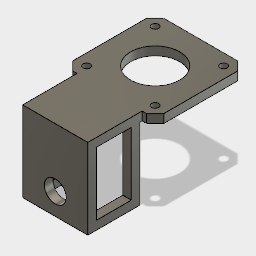
Stepper v4 (Autodesk Fusion 360 design; units mm, degrees)
Autodesk Fusion 360 part; units mm, degrees
note: some values were not read from the file. Set by a fixed rule: which face or edge a step refers to.
sketch "Sketch1" plane through (0, 0, 0) normal (0, 1, 0) x (1, 0, 0)
  line L0 (0, 0) -> (42, 0)
  line L1 (42, 0) -> (42, -42)
  line L2 (42, -42) -> (0, -42)
  line L3 (0, -42) -> (0, 0)
  dimension "d1" = 42
  dimension "d2" = 42
  measures "d1" distance of L0.start L2.end
  measures "d2" distance of L0.start L0.end
extrude "Extrude1" add sketch "Sketch1" along normal blind 33 makes body 1
sketch "Sketch2" plane through (0, 33, 0) normal (0, 1, 0) x (-1, 0, 0)
  line L0 (0, 42) -> (-42, 42)
  line L1 (-42, 42) -> (-42, 0)
  line L2 (-42, 0) -> (0, 0)
  line L3 (0, 0) -> (0, 42)
  circle A0 centre (-21, 21) radius 11.25
  line L4 (-42, 0) -> (-36.75, 0)
  line L5 (-36.75, 0) -> (-36.75, 5.25)
  line L6 (0, 0) -> (-5.25, 0)
  line L7 (-5.25, 0) -> (-5.25, 5.25)
  line L8 (0, 42) -> (-5.25, 42)
  line L9 (-5.25, 42) -> (-5.25, 36.75)
  line L10 (-42, 42) -> (-36.75, 42)
  line L11 (-36.75, 42) -> (-36.75, 36.75)
  circle A1 centre (-5.25, 5.25) radius 1.625
  circle A2 centre (-5.25, 36.75) radius 1.625
  circle A3 centre (-36.75, 36.75) radius 1.625
  circle A4 centre (-36.75, 5.25) radius 1.625
  dimension "d5" = 22.5
  dimension "d15" = 5.25
  dimension "d16" = 5.25
  dimension "d17" = 5.25
  dimension "d18" = 5.25
  dimension "d19" = 5.25
  dimension "d20" = 5.25
  dimension "d21" = 5.25
  dimension "d22" = 5.25
  dimension "d23" = 3.25
  dimension "d24" = 3.25
  dimension "d25" = 3.25
  dimension "d26" = 3.25
  measures "d5" diameter of A0
  measures "d15" distance of L1.end L4.end
  measures "d16" distance of L4.end L5.end
  measures "d17" distance of L2.end L6.end
  measures "d18" distance of L6.end L7.end
  measures "d19" distance of L0.start L8.end
  measures "d20" distance of L8.end L9.end
  measures "d21" distance of L0.end L10.end
  measures "d22" distance of L10.end L11.end
  measures "d23" diameter of A1
  measures "d24" diameter of A2
  measures "d25" diameter of A3
  measures "d26" diameter of A4
extrude "Extrude5" cut sketch "Sketch2" against normal blind 5 contours A1 | A2 | A3 | A4 bodies 1
extrude "Extrude2" add sketch "Sketch2" along normal blind 2 contours A0 bodies 1
sketch "Sketch3" plane through (0, 35, 0) normal (0, 1, 0) x (-1, 0, 0)
  circle A0 centre (-21, 21) radius 11.25
  circle A1 centre (-21, 21) radius 2.5
  dimension "d8" = 5
  measures "d8" diameter of A1
extrude "Extrude3" add sketch "Sketch3" along normal blind 18 contours A1 bodies 1
sketch "Sketch4" plane through (0, 53, 0) normal (0, 1, 0) x (-1, 0, 0)
  circle A0 centre (-21, 21) radius 2.5
  line L0 (-21, 21) -> (-21, 23.5)
  line L1 (-21, 23.5) -> (-21, 19)
  line L2 (-21, 19) -> (-22.5, 19)
  line L3 (-22.5, 19) -> (-19.5, 19)
  dimension "d11" = 90
  measures "d11" angle of L1 L2
extrude "Extrude4" cut sketch "Sketch4" against normal blind 15 contours A0 L2 L3 bodies 1
chamfer "Chamfer1" distance 4 angle 45 4 edges at (42, 16.5, 42) (42, 16.5, 0) (0, 16.5, 42) (0, 16.5, 0) on bodies 1
sketch "Sketch7" plane through (0, 33, 0) normal (0, 1, 0) x (-1, 0, 0)
  line L0 (-4, 0) -> (0, 4)
  line L1 (0, 4) -> (0, 38)
  line L2 (0, 38) -> (-4, 42)
  line L3 (-4, 42) -> (-38, 42)
  line L4 (-38, 42) -> (-42, 38)
  line L5 (-42, 38) -> (-42, 4)
  line L6 (-42, 4) -> (-38, 0)
  line L7 (-38, 0) -> (-4, 0)
  circle A0 centre (-21, 21) radius 11.25
  circle A1 centre (-5.25, 5.25) radius 1.625
  circle A2 centre (-5.25, 36.75) radius 1.625
  circle A3 centre (-36.75, 5.25) radius 1.625
  circle A4 centre (-36.75, 36.75) radius 1.625
  line L8 (0, 42) -> (-42, 42)
  line L9 (-42, 42) -> (-42, 0)
  line L10 (-42, 0) -> (0, 0)
  line L11 (0, 0) -> (0, 42)
  line L12 (0, 42) -> (-42, 0) construction
  line L13 (-42, 42) -> (0, 0) construction
  point P0 (-21, 21)
extrude "Extrude6" add sketch "Sketch7" along normal blind 4 separate body contours L0 L1 L2 L3 L4 L5 L6 L7 L8 L9 L10 L11 makes body 2
sketch "Sketch8" plane through (0, 0, 0) normal (0, 0, 1) x (1, 0, 0)
  circle A0 centre (-30, 0) radius 5
  dimension "d33" = 10
  measures "d33" diameter of A0
extrude "Extrude7" add sketch "Sketch8" along normal blind 100 separate body makes body 3
move_body "Align1" bodies 3 to x (1, 0, 0) y (0, 1, 0) z (0, 0, 1) at (51, 16.5, -58)
move_body "Move1" bodies 3 to x (1, 0, 0) y (0, 1, 0) z (0, 0, 1) at (0, 0, 120)
move_body "Align2" bodies 3 to x (1, 0, 0) y (0, 1, 0) z (0, 0, 1) at (0, 0, -20)
move_body "Move2" bodies 3 to x (1, 0, 0) y (0, 1, 0) z (0, 0, 1) at (0, -5.5, 0)
move_body "Move3" bodies 3 to x (1, 0, 0) y (0, 1, 0) z (0, 0, 1) at (0, -1, 0)
move_body "Move4" bodies 3 to x (1, 0, 0) y (0, 1, 0) z (0, 0, 1) at (0, 0, 10)
move_body "Move5" bodies 1 to x (1, 0, 0) y (0, 1, 0) z (0, 0, 1) at (0, -5, 0)
sketch "Sketch10" plane through (0, 0, 42) normal (0, 0, 1) x (1, 0, 0)
  line L0 (4, 33) -> (38, 33)
  line L1 (38, 33) -> (38, 37)
  line L2 (38, 37) -> (4, 37)
  line L3 (4, 37) -> (4, 33)
  line L4 (36, 33) -> (6, 33)
  line L5 (6, 33) -> (6, 37)
  line L6 (6, 37) -> (36, 37)
  line L7 (36, 37) -> (36, 33)
  line L8 (36, 33) -> (6, 37) construction
  line L9 (6, 33) -> (36, 37) construction
  point P0 (21, 35)
extrude "Extrude8" add sketch "Sketch10" along normal blind 25 contours L0 L2 L4 L5 L6 L7 bodies 2
sketch "Sketch11" plane through (0, 33, 0) normal (0, -1, 0) x (1, 0, 0)
  circle A0 centre (36.75, 36.75) radius 1.625
  circle A1 centre (5.25, 36.75) radius 1.625
  circle A2 centre (21, 21) radius 11.25
  circle A3 centre (36.75, 5.25) radius 1.625
  circle A4 centre (5.25, 5.25) radius 1.625
  line L0 (0, 4) -> (4, 0)
  line L1 (4, 0) -> (38, 0)
  line L2 (38, 0) -> (42, 4)
  line L3 (42, 4) -> (42, 38)
  line L4 (42, 38) -> (38, 42)
  line L5 (38, 42) -> (36, 42)
  line L6 (36, 42) -> (36, 67)
  line L7 (36, 67) -> (6, 67)
  line L8 (6, 67) -> (6, 42)
  line L9 (6, 42) -> (4, 42)
  line L10 (4, 42) -> (0, 38)
  line L11 (0, 38) -> (0, 4)
  line L12 (6, 67) -> (36, 67)
  line L13 (36, 67) -> (36, 63)
  line L14 (36, 63) -> (6, 63)
  line L15 (6, 63) -> (6, 67)
move_body "Move6" bodies 3 to x (1, 0, 0) y (0, 1, 0) z (0, 0, 1) at (0, 0, 29)
extrude "Extrude9" add sketch "Sketch11" along normal blind 35 contours L6 L7 L8 L12 L13 L14 L15 bodies 2
move_body "Move7" bodies 1 to x (1, 0, 0) y (0, 1, 0) z (0, 0, 1) at (0, 0, -5)
sketch "Sketch12" plane through (0, 0, 63) normal (0, 0, -1) x (-1, 0, 0)
  line L0 (-6, 33) -> (-36, 33)
  line L1 (-36, 33) -> (-36, -2)
  line L2 (-36, -2) -> (-6, -2)
  line L3 (-6, -2) -> (-6, 33)
  line L4 (-6, -2) -> (-10, -2)
  line L5 (-10, -2) -> (-10, 2)
  line L6 (-10, 2) -> (-6, 2)
  line L7 (-6, 2) -> (-6, -2)
  line L8 (-36, -2) -> (-32, -2)
  line L9 (-32, -2) -> (-32, 2)
  line L10 (-32, 2) -> (-36, 2)
  line L11 (-36, 2) -> (-36, -2)
  dimension "d42" = 4
  dimension "d43" = 4
  dimension "d44" = 4
  dimension "d45" = 4
  measures "d42" distance of L2.end L4.end
  measures "d43" distance of L2.end L6.end
  measures "d44" distance of L1.end L10.end
  measures "d45" distance of L1.end L8.end
extrude "Extrude10" add sketch "Sketch12" along normal blind 21 contours L2 L3 L4 L5 L6 L7 | L1 L2 L8 L9 L10 L11 bodies 2
sketch "Sketch13" plane through (0, 2, 0) normal (0, 1, 0) x (-1, 0, 0)
  line L0 (-6, 63) -> (-10, 63)
  line L1 (-10, 63) -> (-10, 42)
  line L2 (-10, 42) -> (-6, 42)
  line L3 (-6, 42) -> (-6, 63)
  line L4 (-6, 42) -> (-10, 42)
  line L5 (-10, 42) -> (-10, 46)
  line L6 (-10, 46) -> (-6, 46)
  line L7 (-6, 46) -> (-6, 42)
  line L8 (-32, 42) -> (-36, 42)
  line L9 (-36, 42) -> (-36, 46)
  line L10 (-36, 46) -> (-32, 46)
  line L11 (-32, 46) -> (-32, 42)
  dimension "d48" = 4
  dimension "d49" = 4
  dimension "d50" = 4
  dimension "d51" = 4
  measures "d48" distance of L2.end L1.end
  measures "d49" distance of L2.end L6.end
  measures "d50" distance of L8.start L8.end
  measures "d51" distance of L8.start L10.end
extrude "Extrude11" add sketch "Sketch13" along normal blind 32 contours L1 L2 L3 L4 L5 L6 L7 | L8 L9 L10 L11 bodies 2
move_body "Move8" bodies 1 to x (1, 0, 0) y (0, 1, 0) z (0, 0, 1) at (0, 5, 5)
move_face "OffsetFaces1" offset -2 1 faces at (24.6667, -2, 65.6667) on bodies 2
move_face "OffsetFaces2" offset 2 1 faces at (33.3333, 2, 57.3333) on bodies 2
move_face "OffsetFaces3" offset 2 1 faces at (7.3333, 2, 57.3333) on bodies 2
move_body "Move9" bodies 3 to x (1, 0, 0) y (0, 1, 0) z (0, 0, 1) at (0, 0, -25)
combine "Combine1" operation cut target body 2 tool bodies 3 keep tools
move_face "OffsetFaces4" offset -1 1 faces at (8.6667, 22, 42) on bodies 2
move_face "OffsetFaces5" offset -1 2 faces at (33.3333, 0.6667, 42) (33.3333, 22.6667, 42) on bodies 2
move_face "OffsetFaces6" offset 1 1 faces at (33.3333, 23.3333, 46) on bodies 2
move_face "OffsetFaces7" offset 1 1 faces at (8.6667, 13.6667, 46) on bodies 2
sketch "Sketch14" plane through (0, 53, 0) normal (0, 1, 0) x (-1, 0, 0)
  line L0 (-22.5, 19) -> (-19.5, 19)
  arc A0 (-19.5, 19) -> (-22.5, 19) centre (-21, 21) ccw
  line L1 (0, 0) -> (-42, 0)
  line L2 (-42, 0) -> (-42, 42)
  line L3 (-42, 42) -> (0, 42)
  line L4 (0, 42) -> (0, 0)
sketch "Top View Dimensions" plane through (0, 53, 0) normal (0, 1, 0) x (-1, 0, 0)
  line L0 (-22.5, 19) -> (-19.5, 19)
  arc A0 (-19.5, 19) -> (-22.5, 19) centre (-21, 21) ccw
  line L1 (-4, 0) -> (-38, 0)
  line L2 (0, 0) -> (-42, 0)
  line L3 (-42, 0) -> (-42, 42)
  circle A1 centre (-5.25, 5.25) radius 1.625
  circle A2 centre (-5.25, 5.25) radius 1.625
  line L4 (-5.25, 5.25) -> (-5.25, 0)
  line L5 (0, 38) -> (0, 4)
  line L6 (-5.25, 5.25) -> (0, 5.25)
  circle A3 centre (-21, 21) radius 11.25
  circle A4 centre (-21, 21) radius 11.25
  circle A5 centre (-36.75, 5.25) radius 1.625
  circle A6 centre (-36.75, 5.25) radius 1.625
  line L7 (-36, 67) -> (-36, 43)
  line L8 (-36, 42) -> (-36, 67)
  line L9 (-36, 67) -> (-6, 67)
  line L10 (-6, 67) -> (-36, 67)
  point P0 (-6.875, 5.25)
  point P1 (-38.375, 5.25)
  point P2 (-36, 42)
  point P3 (-36, 67)
  point P4 (-6, 67)
  dimension "d61" = 42
  dimension "d62" = 42
  dimension "d64" = 5.25
  dimension "d65" = 5.25
  dimension "d66" = 22.5
  dimension "d67" = 3.25
  dimension "d68" = 25
  dimension "d69" = 30
  measures "d61" distance of L2.start L2.end
  measures "d62" distance of L2.end L3.end
  measures "d64" distance of A1.centre L6.end
  measures "d65" distance of A1.centre L4.end
  measures "d66" diameter of A3
  measures "d67" diameter of A5
  measures "d68" distance of P2 P3
  measures "d69" distance of P3 P4
sketch "Front View Dimensions" plane through (0, 0, 43) normal (0, 0, -1) x (-1, 0, 0)
  line L0 (-10, 0) -> (-6, 0)
  line L1 (-6, 0) -> (-6, 33)
  line L2 (-6, 33) -> (-10, 33)
  line L3 (-6, 33) -> (-10, 33)
  circle A0 centre (-21, 10) radius 5
  circle A1 centre (-21, 10) radius 5
  circle A2 centre (-21, 10) radius 5
  line L4 (-36, 37) -> (-6, 37)
  line L5 (-36, 0) -> (-6, 0)
  line L6 (-21, 10) -> (-21, 0)
  point P0 (-16, 10)
  point P1 (-38, 37)
  point P2 (-4, 37)
  point P3 (-42, 33)
  point P4 (0, 33)
  point P5 (0, 37)
  dimension "d70" = 4
  dimension "d71" = 33
  dimension "d73" = 10
  dimension "d74" = 34
  dimension "d75" = 42
  dimension "d76" = 37
  dimension "d77" = 10
  measures "d70" distance of L1.end L2.end
  measures "d71" distance of L0.end L1.end
  measures "d73" diameter of A0
  measures "d74" distance of P1 P2
  measures "d75" distance of P3 P4
  measures "d76" distance of origin P5
  measures "d77" distance of A0.centre L6.end
sketch "Side View Dimensions" plane through (0, 0, 0) normal (-1, 0, 0) x (0, 0, 1)
  line L0 (4, 33) -> (38, 33)
  line L1 (38, 33) -> (38, 37)
  line L2 (38, 37) -> (4, 37)
  line L3 (4, 37) -> (4, 33)
  line L4 (67, 37) -> (67, 0)
  line L5 (43, 0) -> (43, 33)
  point P0 (0, 37)
  point P1 (67, 37)
  point P2 (42, 37)
  point P3 (47, 33)
  point P4 (63, 33)
  point P5 (67, 0)
  point P6 (0, 33)
  point P7 (43, 33)
  point P8 (43, 0)
  dimension "d78" = 67
  dimension "d79" = 42
  dimension "d80" = 34
  dimension "d81" = 16
  dimension "d82" = 25
  dimension "d83" = 37
  dimension "d84" = 4
  dimension "d85" = 33
  measures "d78" distance of P0 P1
  measures "d79" distance of P0 P2
  measures "d80" distance of L1.end L2.end
  measures "d81" distance of P3 P4
  measures "d82" distance of P1 P2
  measures "d83" distance of P1 P5
  measures "d84" distance of P0 P6
  measures "d85" distance of P7 P8
hidden bodies 1 3
named bodies: "Stepper", "Stepper to Threaded Mount", "M6 Threaded Rod"
